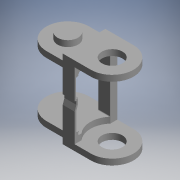
# Autodesk Inventor part: SZ045F-16-018-27c
Saved by Autodesk Inventor 2017.3 (Build 213256000, 256)
## iProperties
Part Number: SZ045F-16-018-27c
Material: Generic
Catalog Web Link: www.cadenas.de
Description: SE08F _ _, SE14F _, SE16F _, SZ08F _ _, SZ14F _, SZ16F _, SE200F _ _,SZ200F _ _, SE300F _ _, SZ300F _ _c-Cable Carriers - Configurable Link Number
Vendor: MISUMI
Document SubType Name: Modeling
Designer: partserver
Manufacturer: MISUMI
Mass: 1.23564 g
Surface Area: 18.022 cm^2
Volume: 1.23564 cm^3
Density: 1 g/cm^3
Appearance: PSOLRGB-192-192-192
Category: PARTsolutions
Company: MISUMI
Title: SZ045F-16-018-27c
Author: Cadenas PARTsolutions
Comments: Cable Carriers - Configurable Link Number
PSOL_IDENT_0: {$CADENAS_DATA\23d-libs\misumi\metric\07_slide_rails\se200f\se08f_clip.prj},290 {VTYP=3D},{NB=SZ045F
PSOL_IDENT_1: -16-018-27c},{LINA=SZ045F-16-018-27c},{NN=SE08F _ _, SE14F _, SE16F _, SZ08F _ _, SZ14F _, SZ16F _,
PSOL_IDENT_2: SE200F _ _,SZ200F _ _, SE300F _ _, SZ300F _ _c},{DATE=30.06.2021 12:54:06},{GEOMDATE=20.09.2012 02:4
PSOL_IDENT_3: 7:00},{VERSION=},{LINEID=40},{WBVAR=TYS,NO,R,NOL},{WBNUMERIC=NO,NOL}  {NB=SZ045F-16-018-27c},{LINA=S
PSOL_IDENT_4: Z045F-16-018-27c},{KT=DUMMY},{PN=SZ045F-16-018-27},{TYPE=SZ045F},{TYS=2},{TYSCONF=045},{TS=SZ045F},{
PSOL_IDENT_5: MAT=Special Plastic},{TU=-30~100},{NO=16},{NO0=16},{STROKE=31},{R=018},{R0='018','028','038'},{R1=18
PSOL_IDENT_6: },{NOL=27},{NOL0=[1-27]},{A=9.4},{B=13.0},{BB=12.5},{C=16},{D=0},{E=0},{W=23.0},{AFFREE=045-16-1},{A
PSOL_IDENT_7: FFIX=045-16-2},{WT=0.11},{H=50},{H1=37.5},{HF=60},{K=95},{DD=50},{P=13.000},{PP=13.0},{HH=12.5},{LL=
PSOL_IDENT_8: 22},{N=4},{LUK=42.33689769166211647},{LUKALT=9.97750},{NALG=25},{T1=2},{T2=3},{K3=42},{K4=32},{K5=42
PSOL_IDENT_9: },{K6=42.336898},{K7=42.336898},{K8=42.336898},{K9=42.336898},{K10=42.336898},{KEND4=31.820858},{KEN
PSOL_IDENT_10: D5=41.798358},{KEND6=31.820858},{KEND7=31.820858},{KEND8=31.820858},{KEND9=31.820858},{KEND10=31.820
PSOL_IDENT_11: 858},{K11=42.336898},{K12=42.336898},{K13=42.336898},{K14=42.336898},{KEND11=31.820858},{KEND12=31.8
PSOL_IDENT_12: 20858},{KEND13=31.820858},{KEND14=31.820858},{KK=31.820858},{KK2=0}
NB: SZ045F-16-018-27c
NN: SE08F _ _, SE14F _, SE16F _, SZ08F _ _, SZ14F _, SZ16F _, SE200F _ _,SZ200F _ _, SE300F _ _, SZ300F _ _c
NT: Cable Carriers - Configurable Link Number
NBSYN: $PN.c
LINA: SZ045F-16-018-27c
CATALOG: Misumi
PN: SZ045F-16-018-27
TYS: Inner Radius Mount Type
TS: SZ045F
MAT: Special Plastic
TU: -30~100
NO: 16
R: 018
NOL: 27
A: 9.4
B: 13
C: 16
D: 0
E: 0
W: 23
WT: 0.11
H: 50
H1: 37.5
HF: 60
K: 95
P: 13
HH: 12.5
LL: 22
SUPPLIER: MISUMI
ARTICLENO: SZ045F-16-018-27c
BOMINFO: SZ045F-16-018-27c
CREATOR: CADENAS GmbH
Autodesk Inventor part; units mm, degrees
sketch "Sketch_1" plane through (0, 0, 0) normal (0, 0, 1) x (1, 0, 0)
  arc A0 (0, 6.25) -> (0, -6.25) centre (0, 0) ccw
  line L0 (0, -6.25) -> (8.25, -6.25)
  line L1 (8.25, -6.25) -> (8.25, -4.2143)
  arc A1 (8.25, 4.2143) -> (8.25, -4.2143) centre (13, 0) ccw
  line L2 (8.25, 4.2143) -> (8.25, 6.25)
  line L3 (8.25, 6.25) -> (0, 6.25)
  circle A2 centre (0, 0) radius 3
  constraints: 8 end point, 4 point on circle, 3 centre point
extrude "Extrusion1" add sketch "Sketch_1" against normal blind 1.75
sketch "Sketch_3" plane through (0, 0, -1.75) normal (0, 0, 1) x (1, 0, 0)
  circle A0 centre (13, 0) radius 3
  constraints: 1 centre point
sketch "Sketch_6" plane through (0, 0, -21.25) normal (0, 0, 1) x (1, 0, 0)
  circle A0 centre (13, 0) radius 3
  constraints: 1 centre point
sketch "Sketch_7" plane through (0, 0, -21.25) normal (0, 0, 1) x (1, 0, 0)
  arc A0 (0, 6.25) -> (0, -6.25) centre (0, 0) ccw
  line L0 (0, -6.25) -> (8.25, -6.25)
  line L1 (8.25, -6.25) -> (8.25, -4.2143)
  arc A1 (8.25, 4.2143) -> (8.25, -4.2143) centre (13, 0) ccw
  line L2 (8.25, 4.2143) -> (8.25, 6.25)
  line L3 (8.25, 6.25) -> (0, 6.25)
  circle A2 centre (0, 0) radius 3
  constraints: 8 end point, 4 point on circle, 3 centre point
sketch "Sketch_4" plane through (0, 0, -19.5) normal (0, 0, 1) x (1, 0, 0)
  line L0 (4.75, 6.25) -> (4.75, -6.25)
  line L1 (4.75, -6.25) -> (13, -6.25)
  arc A0 (13, -6.25) -> (13, 6.25) centre (13, 0) ccw
  line L2 (13, 6.25) -> (4.75, 6.25)
  constraints: 6 end point, 2 point on circle, 1 centre point
sketch "Sketch_5" plane through (0, 0, -1.75) normal (0, 0, 1) x (1, 0, 0)
  line L0 (4.75, 6.25) -> (4.75, -6.25)
  line L1 (4.75, -6.25) -> (13, -6.25)
  arc A0 (13, -6.25) -> (13, 6.25) centre (13, 0) ccw
  line L2 (13, 6.25) -> (4.75, 6.25)
  constraints: 6 end point, 2 point on circle, 1 centre point
extrude "Extrusion2" add sketch "Sketch_5" against normal blind 1.75
extrude "Extrusion3" add sketch "Sketch_3" along normal blind 1.75
sketch "Sketch_9" plane through (6.5, 0, 0) normal (1, 0, 0) x (0, 0, -1)
  arc A0 (3.7, 4.173) -> (3.5, 3.973) centre (3.7, 3.973) ccw
  line L0 (3.7, 4.173) -> (19.3, 4.173)
  arc A1 (19.5, 3.973) -> (19.3, 4.173) centre (19.3, 3.973) ccw
  line L1 (19.5, 3.973) -> (19.5, 6.25)
  line L2 (19.5, 6.25) -> (3.5, 6.25)
  line L3 (3.5, 6.25) -> (3.5, 3.973)
  constraints: 8 end point, 4 point on circle, 2 centre point
extrude "Extrusion4" add sketch "Sketch_9" along normal mid plane 3.5
sketch "Sketch_11" plane through (6.5, 0, 0) normal (1, 0, 0) x (0, 0, -1)
  line L0 (3.5, -5.0148) -> (3.5, -6.25)
  line L1 (3.5, -6.25) -> (10, -6.25)
  line L2 (10, -6.25) -> (11.5, -5.7333)
  line L3 (11.5, -5.7333) -> (13, -5.7333)
  arc A0 (13, -5.2167) -> (13, -5.7333) centre (13.2583, -5.475) ccw
  line L4 (13, -5.2167) -> (11.5, -5.2167)
  line L5 (11.5, -5.2167) -> (10, -5.7333)
  line L6 (10, -5.7333) -> (4.7, -5.7333)
  arc A1 (4.5, -5.5333) -> (4.7, -5.7333) centre (4.7, -5.5333) ccw
  line L7 (4.5, -5.5333) -> (4.5, -4.9347)
  arc A2 (3.5, -5.0148) -> (4.5, -4.9347) centre (3.97, -4.6003) ccw
  constraints: 16 end point, 6 point on circle, 3 centre point
extrude "Extrusion5" add sketch "Sketch_11" along normal mid plane 3.5
sketch "Sketch_12" plane through (6.5, 0, 0) normal (1, 0, 0) x (0, 0, -1)
  line L0 (12.5, -5.8071) -> (12.5, -5.95)
  arc A0 (12.5, -5.95) -> (12.8, -6.25) centre (12.8, -5.95) ccw
  line L1 (12.8, -6.25) -> (19.5, -6.25)
  line L2 (19.5, -6.25) -> (19.5, -4.6689)
  arc A1 (18.5, -5.227) -> (19.5, -4.6689) centre (18.5, -4.052) ccw
  line L3 (18.5, -5.227) -> (18.5, -5.6071)
  arc A2 (18.3, -5.8071) -> (18.5, -5.6071) centre (18.3, -5.6071) ccw
  line L4 (18.3, -5.8071) -> (13.049, -5.8071)
  arc A3 (12.9618, -5.7915) -> (13.049, -5.8071) centre (13.049, -5.5571) ccw
  arc A4 (12.9618, -5.7915) -> (12.5, -5.8071) centre (12.75, -6.361) ccw
  constraints: 10 end point, 10 point on circle, 5 centre point
extrude "Extrusion6" add sketch "Sketch_4" against normal blind 1.75
extrude "Extrusion7" add sketch "Sketch_6" against normal blind 1.75
extrude "Extrusion8" add sketch "Sketch_7" against normal blind 1.75
extrude "Extrusion9" add sketch "Sketch_12" along normal mid plane 3.5
sketch "Sketch_19" plane through (0, 0, -1.75) normal (0, 0, 1) x (1, 0, 0)
  line L0 (-8.25, 6.35) -> (-8.25, -6.35)
  line L1 (-8.25, -6.35) -> (0, -6.35)
  arc A0 (0, -6.35) -> (0, 6.35) centre (0, 0) ccw
  line L2 (0, 6.35) -> (-8.25, 6.35)
  constraints: 6 end point, 2 point on circle, 1 centre point
extrude "Extrusion10" cut sketch "Sketch_19" against normal blind 9.75
sketch "Sketch_20" plane through (0, 0, -21.25) normal (0, 0, 1) x (1, 0, 0)
  line L0 (-8.25, 6.35) -> (-8.25, -6.35)
  line L1 (-8.25, -6.35) -> (0, -6.35)
  arc A0 (0, -6.35) -> (0, 6.35) centre (0, 0) ccw
  line L2 (0, 6.35) -> (-8.25, 6.35)
  constraints: 6 end point, 2 point on circle, 1 centre point
extrude "Extrusion11" cut sketch "Sketch_20" along normal blind 9.75
ref_plane "R1_XY" through (0, 0, 0) normal (0, 0, 1) x (1, 0, 0)
ref_plane "R1_YZ" through (0, 0, 0) normal (1, 0, 0) x (0, 1, 0)
ref_plane "R1_ZX" through (0, 0, 0) normal (0, 1, 0) x (0, 0, 1)
ref_plane "clip_to_dummy_XY" through (6.5, -18, -11.5) normal (0, 0, 1) x (1, 0, 0)
ref_plane "clip_to_dummy_YZ" through (6.5, -18, -11.5) normal (1, 0, 0) x (0, 1, 0)
ref_plane "clip_to_dummy_ZX" through (6.5, -18, -11.5) normal (0, 1, 0) x (0, 0, 1)
ref_plane "move_1_XY" through (13, 0, 0) normal (0, 0, 1) x (1, 0, 0)
ref_plane "move_1_YZ" through (13, 0, 0) normal (1, 0, 0) x (0, 1, 0)
ref_plane "move_1_ZX" through (13, 0, 0) normal (0, 1, 0) x (0, 0, 1)
ref_plane "move_2_XY" through (0, 0, 0) normal (0, 0, 1) x (1, 0, 0)
ref_plane "move_2_YZ" through (0, 0, 0) normal (1, 0, 0) x (0, 1, 0)
ref_plane "move_2_ZX" through (0, 0, 0) normal (0, 1, 0) x (0, 0, 1)
ref_plane "move_end_XY" through (13, 0, 0) normal (0, 0, 1) x (1, 0, 0)
ref_plane "move_end_YZ" through (13, 0, 0) normal (1, 0, 0) x (0, 1, 0)
ref_plane "move_end_ZX" through (13, 0, 0) normal (0, 1, 0) x (0, 0, 1)
body "Solid1"
